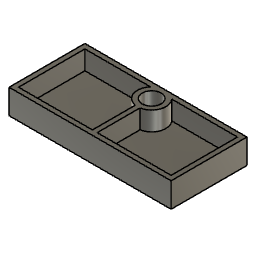
Reservoir Tanks (Autodesk Fusion 360 design; units mm, degrees)
Autodesk Fusion 360 part; units mm, degrees
sketch "Sketch1" plane through (0, 0, 0) normal (0, 0, 1) x (1, 0, 0)
  line L0 (0, 0) -> (171, 0)
  line L1 (171, 0) -> (171, 80)
  line L2 (171, 80) -> (0, 80)
  line L3 (0, 80) -> (0, 0)
  dimension "d1" = 171
  dimension "d2" = 80
  constraint horizontal L0
  constraint vertical L1
  constraint horizontal L2
  constraint vertical L3
  constraint coincident L0.start L3.end
  measures "d1" distance of L1 L3
  measures "d2" distance of L0 L2
extrude "Extrude1" add sketch "Sketch1" along normal blind 59
sketch "Sketch2" plane through (0, 0, 59) normal (0, 0, 1) x (-1, 0, 0)
  line L0 (0, -80) -> (0, 0)
  line L1 (0, 0) -> (-171, 0)
  line L2 (-171, 0) -> (-171, -80)
  line L3 (-171, -80) -> (0, -80)
  line L4 (-166, -5) -> (-88, -5)
  line L5 (-88, -5) -> (-88, -75)
  line L6 (-88, -75) -> (-166, -75)
  line L7 (-166, -75) -> (-166, -5)
  line L8 (-85.5, 0) -> (-85.5, -80)
  line L9 (-5, -5) -> (-83, -5)
  line L10 (-5, -75) -> (-5, -5)
  line L11 (-83, -5) -> (-83, -75)
  line L12 (-83, -75) -> (-5, -75)
  dimension "d5" = 85.5
  dimension "d6" = 70
  dimension "d8" = 5
  dimension "d9" = 5
  dimension "d10" = 2.5
  dimension "d11" = 5
  constraint horizontal L4
  constraint vertical L5
  constraint horizontal L6
  constraint vertical L7
  constraint midpoint L1 L8.start
  constraint midpoint L3 L8.end
  constraint symmetric L4.start L8 L9.start
  constraint symmetric L4.end L8 L9.end
  constraint symmetric L5.end L8 L11.end
  constraint symmetric L6.end L8 L10.start
  measures "d5" distance of L0 L8
  measures "d6" distance of L4.end L5.end
  measures "d8" distance of L3 L6
  measures "d9" distance of L2 L7
  measures "d10" distance of L5 L8
  measures "d11" distance of L1 L4
extrude "Extrude2" cut sketch "Sketch2" against normal blind 10 contours L4 L5 L6 L7 | L9 L10 L11 L12
extrude "Extrude3" cut 2 faces at (57, 28.3333, 49) (140, 28.3333, 49) along direction (0, 0, -1) blind 10
sketch "Sketch3" plane through (0, 0, 59) normal (0, 0, 1) x (-1, 0, 0)
  line L0 (-88, -5) -> (-88, -75)
  line L1 (-88, -75) -> (-166, -75)
  line L2 (-166, -75) -> (-166, -5)
  line L3 (-166, -5) -> (-88, -5)
  line L4 (-5, -5) -> (-5, -75)
  line L5 (-5, -75) -> (-83, -75)
  line L6 (-83, -75) -> (-83, -5)
  line L7 (-83, -5) -> (-5, -5)
  line L8 (0, -80) -> (0, 0)
  line L9 (0, 0) -> (-171, 0)
  line L10 (-171, 0) -> (-171, -80)
  line L11 (-171, -80) -> (0, -80)
  circle A0 centre (-85.5, -65) radius 10
  line L12 (-85.5, 0) -> (-85.5, -80)
  line L13 (-83, -75) -> (-5, -75)
  circle A1 centre (-85.5, -65) radius 15
  dimension "d16" = 20
  dimension "d17" = 10
  dimension "d18" = 30
  constraint coincident A0.centre L12
  constraint concentric A0 A1
  measures "d16" diameter of A0
  measures "d17" distance of A0.centre L13
  measures "d18" diameter of A1
extrude "Extrude4" add sketch "Sketch3" against normal blind 20 contours L0 L1 A0 A1 | L5 L6 A0 L13 A1
extrude "Extrude5" cut sketch "Sketch3" against normal blind 20 contours L0 A0 L12 | L6 A0 L12
sketch "Sketch4" plane through (0, 0, 0) normal (0, -1, 0) x (1, 0, 0)
  line L0 (0, 0) -> (171, 0)
  line L1 (171, 0) -> (171, 59)
  line L2 (171, 59) -> (0, 59)
  line L3 (0, 59) -> (0, 0)
  line L4 (0, 0) -> (171, 0)
  line L5 (171, 0) -> (171, 30)
  line L6 (171, 30) -> (0, 30)
  line L7 (0, 30) -> (0, 0)
  dimension "d23" = 30
  constraint horizontal L4
  constraint vertical L5
  constraint horizontal L6
  constraint vertical L7
  constraint coincident L0.start L3.end
  measures "d23" distance of L4 L6
extrude "Extrude6" cut sketch "Sketch4" against normal blind 80 contours L0 L1 L3 L4 L5 L6 L7
sketch "Sketch5" plane through (0, 0, 30) normal (0, 0, -1) x (1, 0, 0)
  line L0 (171, 0) -> (0, 0)
  line L1 (0, 0) -> (0, -80)
  line L2 (0, -80) -> (171, -80)
  line L3 (171, -80) -> (171, 0)
  line L4 (166, -75) -> (5, -75)
  line L5 (5, -75) -> (5, -5)
  line L6 (5, -5) -> (166, -5)
  line L7 (166, -5) -> (166, -75)
  point P0 (166, -75)
  point P1 (5, -5)
  constraint horizontal L4
  constraint vertical L5
  constraint horizontal L6
  constraint vertical L7
  constraint coincident P1 L5.end
  constraint coincident P0 L4.start
extrude "Extrude7" cut sketch "Sketch5" against normal blind 3
